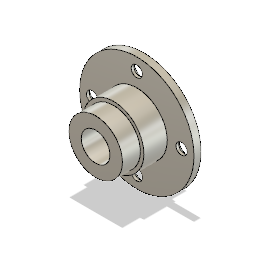
sun_gear_holder_38_20190404 (Autodesk Fusion 360 design; units mm, degrees)
Autodesk Fusion 360 part; units mm, degrees
sketch "Outer Ring" plane through (0, 0, 0) normal (0, 0, 1) x (1, 0, 0)
  circle A0 centre (0, 0) radius 16
  dimension "d359" = 32
  dimension "d387" = 0
  dimension "d388" = 0
  dimension "d389" = 0
  dimension "d390" = 0
  dimension "d493" = 0
  dimension "d494" = 0
  dimension "d495" = 0
  dimension "d496" = 0
  dimension "d520" = 0
  dimension "d521" = 0
  dimension "d522" = 0
  dimension "d523" = 0
  dimension "d532" = 0
  dimension "d533" = 0
  dimension "d534" = 0
  dimension "d535" = 0
  dimension "d830" = 0
  dimension "d831" = 0
  dimension "d832" = 0
  dimension "d833" = 0
  measures "d359" diameter of A0
extrude "Extrude1" add sketch "Outer Ring" against normal blind 2
sketch "Housing Bearing Lip" plane through (0, 0, -2) normal (0, 0, -1) x (-1, 0, 0)
  circle A0 centre (0, 0) radius 16
  circle A1 centre (0, 0) radius 8.5
  dimension "d360" = 17
  measures "d360" diameter of A1
extrude "Extrude2" add sketch "Housing Bearing Lip" along normal blind 0.5 contours A1
sketch "Housing Bearing Stud" plane through (0, 0, -2.5) normal (0, 0, -1) x (-1, 0, 0)
  circle A0 centre (0, 0) radius 8.5
  circle A1 centre (0, 0) radius 7.5
  dimension "d363" = 15
  measures "d363" diameter of A1
extrude "Extrude3" add sketch "Housing Bearing Stud" along normal blind 4.1 contours A1
sketch "Sketch4" plane through (0, 0, 0) normal (0, 0, 1) x (1, 0, 0)
  circle A0 centre (0, 0) radius 16
  circle A1 centre (0, 0) radius 7.5
  circle A2 centre (0, 0) radius 6.375
  dimension "d386" = 15
  measures "d386" diameter of A1
extrude "Extrude4" add sketch "Sketch4" along normal blind 11.5 contours A1 | A2
sketch "Sun Gear Cavity" plane through (0, 0, 11.5) normal (0, 0, 1) x (1, 0, 0)
  circle A0 centre (0, 0) radius 4
  circle A1 centre (0, 0) radius 7.5
  dimension "d368" = 8
  measures "d368" diameter of A0
extrude "Extrude5" cut sketch "Sun Gear Cavity" against normal blind 12 contours A0
sketch "Position Magnet Cavity" plane through (0, 0, -6.6) normal (0, 0, -1) x (-1, 0, 0)
  circle A0 centre (0, 0) radius 7.5
  circle A1 centre (0, 0) radius 3.2385
  dimension "d371" = 6.477
  measures "d371" diameter of A1
extrude "Extrude6" cut sketch "Position Magnet Cavity" against normal blind 3.2 contours A1
sketch "Planet Input Bearing Lip" plane through (0, 0, 0) normal (0, 0, 1) x (1, 0, 0)
  circle A0 centre (0, 0) radius 7.5
  circle A1 centre (0, 0) radius 16
  circle A2 centre (0, 0) radius 8.5
  dimension "d399" = 17
  measures "d399" diameter of A2
extrude "Extrude7" add sketch "Planet Input Bearing Lip" along normal blind 6.5 contours A2
sketch "RotorMountHoles" plane through (0, 0, -2) normal (0, 0, -1) x (-1, 0, 0)
  circle A0 centre (0, 0) radius 8.5
  circle A1 centre (0, 0) radius 16
  circle A2 centre (0, 12.5) radius 1.5
  circle A3 centre (12.5, 0) radius 1.5
  circle A4 centre (0, -12.5) radius 1.5
  circle A5 centre (-12.5, 0) radius 1.5
  circle A6 centre (0, 12.5) radius 1.55
  circle A7 centre (12.5, 0) radius 1.55
  circle A8 centre (0, -12.5) radius 1.55
  circle A9 centre (-12.5, 0) radius 1.55
  dimension "d402" = 3.1
  measures "d402" diameter of A9
hole "Hole1" at (0, 12.5, -2) at (-12.5, 0, -2) at (0, -12.5, -2) at (12.5, 0, -2) direction (0, 0, 1) diameter 3.1 depth 5 tip angle 118 countersink diameter 5.6 countersink angle 90
sketch "CentralPinHole" plane through (0, 0, 0) normal (0, 0, 1) x (1, 0, 0)
  circle A0 centre (0, 0) radius 2.1
  dimension "d694" = 4.2
  measures "d694" diameter of A0
extrude "Extrude9" cut sketch "CentralPinHole" along normal mid plane 40
equation "d360 = RotorBearingID + 2 mm"
equation "d363 = RotorBearingID"
equation "d364 = RotorBearingWidth + 0.1 mm"
equation "d371 = 6.35 mm + 0.127 mm"
equation "d386 = InputBearingID"
equation "d399 = InputBearingID + 2 mm"
equation "InputBearingID = 15 mm"
equation "RotorBearingID = 15 mm"
equation "RotorBearingWidth = 4 mm"
